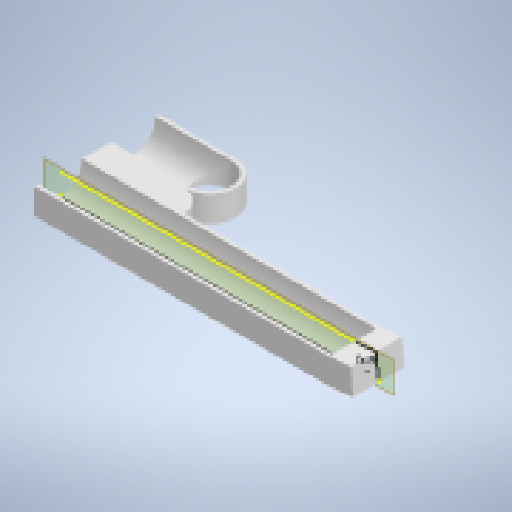
# Autodesk Inventor part: Pega uma e libera menor
Saved by Autodesk Inventor 2024 (Build 280153000, 153)
## iProperties
Created: 2023-05-16
Part Number: Pega uma e libera menor
Material: Genérico
Document SubType Name: Modeling
Designer: jpjoa
Density: 1 g/cm^3
Appearance: Padrão
Author: jpjoa
Autodesk Inventor part; units mm, degrees
ref_plane "YZ Plane" through (0, 0, 0) normal (1, 0, 0) x (0, 1, 0)
ref_plane "XZ Plane" through (0, 0, 0) normal (0, 1, 0) x (-1, 0, 0)
ref_plane "XY Plane" through (0, 0, 0) normal (0, 0, 1) x (1, 0, 0)
sketch "Esboço1" plane through (0, 0, 0) normal (0, 1, 0) x (-1, 0, 0)
  line L0 (0, -1.6) -> (-121.2934, -1.6)
  line L1 (-121.2934, -19.6) -> (0, -19.6)
  circle A0 centre (-31.4625, -40.8) radius 9
  line L2 (-31.4625, -31.8) -> (0, -31.8)
  line L3 (0, -49.8) -> (-31.4625, -49.8)
  arc A1 (-31.4625, -30.2) -> (-31.4625, -51.4) centre (-31.4625, -40.8) ccw
  line L4 (-31.4625, -51.4) -> (0, -51.4)
  line L5 (0, -51.4) -> (0, -31.8)
  line L6 (0, -21.2) -> (0, 0)
  line L7 (0, 0) -> (-121.2934, 0)
  line L8 (-121.2934, 0) -> (-121.2934, -21.2)
  line L9 (-121.2934, -21.2) -> (0, -21.2)
  line L10 (0, -30.2) -> (-31.4625, -30.2)
  line L11 (0, -21.2) -> (0, -30.2)
  line L12 (0, -30.2) -> (0, -31.8)
  arc A2 (-40.4625, -21.2) -> (-31.4625, -30.2) centre (-31.4625, -21.2) ccw
  line L13 (-31.4625, -30.2) -> (-31.4625, -21.2) construction
  line L14 (-40.4625, -21.2) -> (-31.4625, -21.2) construction
  point P0 (-40.4625, -21.2)
  point P1 (0, -31.8)
  dimension "d0" = 18
  dimension "d2" = 1.6
  dimension "d3" = 1.6
  dimension "d4" = 1.6
  dimension "d6" = 18
  dimension "d7" = 1.6
  dimension "d8" = 9
  dimension "d9" = 90
  constraints: 30 end point, 6 point on circle, 6 point on line, 4 horizontal, 4 perpendicular, 3 centre point, 3 coincident, 3 tangent, 2 vertical, 1 horizontal alignment, 1 vertical alignment
  measures "d0" diameter of A0
  measures "d2" radial gap between concentric circles of A0 A1
  measures "d3" distance between parallel lines of L3 L4
  measures "d4" distance between parallel lines of L1 L9
  measures "d6" distance between parallel lines of L0 L1
  measures "d7" distance between parallel lines of L7 L0
  measures "d8" distance of L6.start L10.start
  measures "d9" angle of L14 L13
extrude "Extrusão1" add sketch "Esboço1" against normal blind 1.6 contours L6 L1 L8 L0 | L0 L8 L7 L6 | L6 L9 L8 L1 | L11 L10 A2 L9 | L12 L2 A0 L3 L5 L4 A1 L10 | L5 L3 A0 L2
extrude "Extrusão2" add sketch "Esboço1" along normal blind 9 contours L0 L8 L7 L6 | L6 L9 L8 L1 | L11 L10 A2 L9 | L12 L2 A0 L3 L5 L4 A1 L10
fillet "Arredondamento1" radius 9 4 edges at (60.6467, 0, -19.6) (60.6467, 0, -1.6) (15.7312, 0, -31.8) (15.7312, 0, -49.8)
sketch "Esboço4" plane through (0, -1.6, 0) normal (0, 0, 1) x (1, 0, 0)
  line L0 (121.2934, 0) -> (0, 0) projected
  line L1 (121.2934, 0) -> (131.2553, 0.8716)
  line L2 (121.2934, 0) -> (131.2934, 0) construction
  line L3 (131.2553, 0.8716) -> (130.335, 11.391)
  line L4 (0, 10.6) -> (121.2934, 10.6) projected
  line L5 (130.335, 11.391) -> (121.2934, 10.6)
  line L6 (121.2934, 0) -> (121.2934, 10.6)
  point P0 (0, 1.6)
  dimension "d22" = 10
  dimension "d23" = 5
  constraints: 10 end point, 3 perpendicular, 1 equal length, 1 horizontal
  measures "d22" distance of L0.start L1.end
  measures "d23" angle of L2 L1
extrude "Extrusão5" add sketch "Esboço4" against normal up to surface (21.2 mm away)
ref_plane "Plano de trabalho1" through (40.4625, -1.6, -10.6) normal (0, 0, -1) x (-1, 0, 0)
sketch "Esboço5" plane through (40.4625, -1.6, -10.6) normal (0, 0, -1) x (-1, 0, 0)
  line L0 (-89.8725, 11.391) -> (-80.8309, 10.6) projected
  line L1 (40.4625, 10.6) -> (-80.8309, 10.6) projected
  line L2 (-80.8309, 1.6) -> (40.4625, 1.6)
  line L3 (-90.7928, 0.8716) -> (-89.8725, 11.391) projected
  line L4 (-90.6569, 2.4253) -> (-89.8725, 11.391)
  line L5 (-89.8725, 11.391) -> (-80.8309, 10.6)
  line L6 (-80.8309, 10.6) -> (-80.8309, 1.6) projected
  line L7 (-80.8309, 1.6) -> (-80.8309, 10.6)
  line L8 (-90.6569, 2.4253) -> (-81.2238, 1.6)
  line L9 (-81.2238, 1.6) -> (-80.8309, 1.6)
  point P0 (40.4625, 1.6)
  point P1 (-80.8309, 1.6)
  dimension "d28" = 9.4691
  constraints: 12 end point, 3 collinear, 2 point on line, 1 horizontal, 1 parallel
  measures "d28" distance of L4.start L8.end
extrude "Extrusão6" cut sketch "Esboço5" along normal mid plane 18
fillet "Arredondamento2" radius 9 2 edges at (126.4029, 0.4126, -19.6) (126.4029, 0.4126, -1.6)
equation "\"d0\" = Esfera"
equation "\"d2\" = Margem"
equation "\"d3\" = Margem"
equation "\"d4\" = Margem"
equation "\"d6\" = Esfera"
equation "\"d7\" = Margem"
equation "\"d10\" = Margem"
equation "\"d12\" = 0.5 * Esfera"
equation "\"d14\" = 0.5 * Esfera"
equation "\"d29\" = Esfera"
equation "\"d31\" = 0.5 * Esfera"
equation "\"Esfera\" = 18"
equation "\"Margem\" = 1.6"
